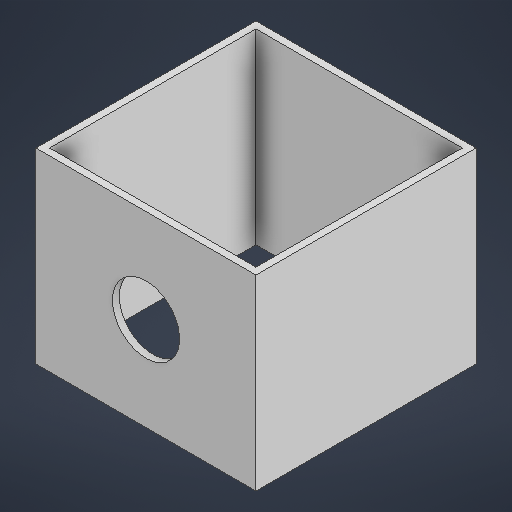
# Autodesk Inventor part: Container
Saved by Autodesk Inventor 2026 (Build 300175050, 175E)
## iProperties
Created: 2025-11-03
Part Number: Container
Material: Generic
Document SubType Name: Modeling
Designer: randy
Density: 1 g/cm^3
Appearance: Default
Author: randy
Autodesk Inventor part; units mm, degrees
ref_plane "YZ Plane" through (0, 0, 0) normal (1, 0, 0) x (0, 1, 0)
ref_plane "XZ Plane" through (0, 0, 0) normal (0, 1, 0) x (-1, 0, 0)
ref_plane "XY Plane" through (0, 0, 0) normal (0, 0, 1) x (1, 0, 0)
sketch "Sketch1" plane through (0, 0, 0) normal (0, 1, 0) x (-1, 0, 0)
  line L0 (-25.4, -25.4) -> (25.4, -25.4)
  line L1 (25.4, -25.4) -> (25.4, 25.4)
  line L2 (25.4, 25.4) -> (-25.4, 25.4)
  line L3 (-25.4, 25.4) -> (-25.4, -25.4)
  line L4 (-25.4, -25.4) -> (25.4, 25.4) construction
  line L5 (25.4, -25.4) -> (-25.4, 25.4) construction
  line L6 (23.8125, 23.8125) -> (23.8125, -23.8125)
  line L7 (23.8125, -23.8125) -> (-23.8125, -23.8125)
  line L8 (-23.8125, -23.8125) -> (-23.8125, 23.8125)
  line L9 (-23.8125, 23.8125) -> (23.8125, 23.8125)
  point P0 (0, 0)
  dimension "d0" = 50.8
  dimension "d1" = 50.8
  dimension "d2" = 1.5875
  constraints: 20 end point, 4 parallel, 2 midpoint, 2 perpendicular, 1 horizontal, 3 other
  measures "d0" distance of L2.end L1.end
  measures "d1" distance of L1.end L0.end
  measures "d2" distance between parallel lines of L1 L6
extrude "Extrusion1" add sketch "Sketch1" along normal mid plane 43.18
sketch "Sketch2" plane through (-25.4, 21.59, 25.4) normal (0, 0, 1) x (1, 0, 0)
  circle A0 centre (25.4, -21.59) radius 7.747
  dimension "d5" = 15.494
  constraints: 1 centre point, 1 coincident
  measures "d5" diameter of A0
extrude "Extrusion2" cut sketch "Sketch2" along normal mid plane 43.18
body "Solid1"
